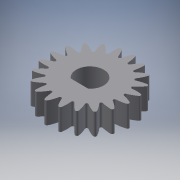
# Autodesk Inventor part: Kugg
Saved by Autodesk Inventor 2016 (Build 200138000, 138)
## iProperties
Created: 2018-03-02
Part Number: Kugg
Material: Generic
Document SubType Name: Modeling
Designer: Simon
Density: 1 g/cm^3
Appearance: Default
Author: Simon
Autodesk Inventor part; units mm, degrees
ref_plane "YZ Plane" through (0, 0, 0) normal (1, 0, 0) x (0, 1, 0)
ref_plane "XZ Plane" through (0, 0, 0) normal (0, 1, 0) x (-1, 0, 0)
ref_plane "XY Plane" through (0, 0, 0) normal (0, 0, 1) x (1, 0, 0)
sketch "Sketch1" plane through (0, 0, 0) normal (0, 0, 1) x (1, 0, 0)
  circle A0 centre (0, 0) radius 5.75
  arc A1 (0.266, 7.6325) -> (-0.3296, 5.7405) centre (6.5778, 4.6059) ccw
  arc A2 (1.143, 5.6352) -> (0.8227, 7.5927) centre (-5.8555, 5.495) ccw
  arc A3 (0.8227, 7.5927) -> (0.266, 7.6325) centre (0.5365, 7.5028) ccw
  arc A4 (-2.1056, 7.3412) -> (-2.0874, 5.3577) centre (4.8326, 6.4131) ccw
  arc A5 (-1.5638, 7.4753) -> (-2.1056, 7.3412) centre (-1.8082, 7.3014) ccw
  arc A6 (-0.6543, 5.7127) -> (-1.5638, 7.4753) centre (-7.267, 3.4166) ccw
  arc A7 (-4.2711, 6.3312) -> (-3.6408, 4.4505) centre (2.6143, 7.5926) ccw
  arc A8 (-3.7973, 6.6262) -> (-4.2711, 6.3312) centre (-3.976, 6.3853) ccw
  arc A9 (-2.3876, 5.2309) -> (-3.7973, 6.6262) centre (-7.9671, 1.0037) ccw
  arc A10 (-6.0185, 4.7015) -> (-4.8379, 3.1076) centre (0.1401, 8.0288) ccw
  arc A11 (-5.659, 5.1285) -> (-6.0185, 4.7015) centre (-5.7545, 4.8441) ccw
  arc A12 (-3.8871, 4.2371) -> (-5.659, 5.1285) centre (-7.8873, -1.5074) ccw
  arc A13 (-7.1768, 2.6116) -> (-5.5614, 1.4605) centre (-2.3478, 7.6792) ccw
  arc A14 (-6.9669, 3.1287) -> (-7.1768, 2.6116) centre (-6.9698, 2.8288) ccw
  arc A15 (-5.0062, 2.8285) -> (-6.9669, 3.1287) centre (-7.0355, -3.8709) ccw
  arc A16 (-7.6325, 0.266) -> (-5.7405, -0.3296) centre (-4.6059, 6.5778) ccw
  arc A17 (-7.5927, 0.8227) -> (-7.6325, 0.266) centre (-7.5028, 0.5365) ccw
  arc A18 (-5.6352, 1.143) -> (-7.5927, 0.8227) centre (-5.495, -5.8555) ccw
  arc A19 (-7.3412, -2.1056) -> (-5.3577, -2.0874) centre (-6.4131, 4.8326) ccw
  arc A20 (-7.4753, -1.5638) -> (-7.3412, -2.1056) centre (-7.3014, -1.8082) ccw
  arc A21 (-5.7127, -0.6543) -> (-7.4753, -1.5638) centre (-3.4166, -7.267) ccw
  arc A22 (-6.3312, -4.2711) -> (-4.4505, -3.6408) centre (-7.5926, 2.6143) ccw
  arc A23 (-6.6262, -3.7973) -> (-6.3312, -4.2711) centre (-6.3853, -3.976) ccw
  arc A24 (-5.2309, -2.3876) -> (-6.6262, -3.7973) centre (-1.0037, -7.9671) ccw
  arc A25 (-4.7015, -6.0185) -> (-3.1076, -4.8379) centre (-8.0288, 0.1401) ccw
  arc A26 (-5.1285, -5.659) -> (-4.7015, -6.0185) centre (-4.8441, -5.7545) ccw
  arc A27 (-4.2371, -3.8871) -> (-5.1285, -5.659) centre (1.5074, -7.8873) ccw
  arc A28 (-2.6116, -7.1768) -> (-1.4605, -5.5614) centre (-7.6792, -2.3478) ccw
  arc A29 (-3.1287, -6.9669) -> (-2.6116, -7.1768) centre (-2.8288, -6.9698) ccw
  arc A30 (-2.8285, -5.0062) -> (-3.1287, -6.9669) centre (3.8709, -7.0355) ccw
  arc A31 (-0.266, -7.6325) -> (0.3296, -5.7405) centre (-6.5778, -4.6059) ccw
  arc A32 (-0.8227, -7.5927) -> (-0.266, -7.6325) centre (-0.5365, -7.5028) ccw
  arc A33 (-1.143, -5.6352) -> (-0.8227, -7.5927) centre (5.8555, -5.495) ccw
  arc A34 (2.1056, -7.3412) -> (2.0874, -5.3577) centre (-4.8326, -6.4131) ccw
  arc A35 (1.5638, -7.4753) -> (2.1056, -7.3412) centre (1.8082, -7.3014) ccw
  arc A36 (0.6543, -5.7127) -> (1.5638, -7.4753) centre (7.267, -3.4166) ccw
  arc A37 (4.2711, -6.3312) -> (3.6408, -4.4505) centre (-2.6143, -7.5926) ccw
  arc A38 (3.7973, -6.6262) -> (4.2711, -6.3312) centre (3.976, -6.3853) ccw
  arc A39 (2.3876, -5.2309) -> (3.7973, -6.6262) centre (7.9671, -1.0037) ccw
  arc A40 (6.0185, -4.7015) -> (4.8379, -3.1076) centre (-0.1401, -8.0288) ccw
  arc A41 (5.659, -5.1285) -> (6.0185, -4.7015) centre (5.7545, -4.8441) ccw
  arc A42 (3.8871, -4.2371) -> (5.659, -5.1285) centre (7.8873, 1.5074) ccw
  arc A43 (7.1768, -2.6116) -> (5.5614, -1.4605) centre (2.3478, -7.6792) ccw
  arc A44 (6.9669, -3.1287) -> (7.1768, -2.6116) centre (6.9698, -2.8288) ccw
  arc A45 (5.0062, -2.8285) -> (6.9669, -3.1287) centre (7.0355, 3.8709) ccw
  arc A46 (7.6325, -0.266) -> (5.7405, 0.3296) centre (4.6059, -6.5778) ccw
  arc A47 (7.5927, -0.8227) -> (7.6325, -0.266) centre (7.5028, -0.5365) ccw
  arc A48 (5.6352, -1.143) -> (7.5927, -0.8227) centre (5.495, 5.8555) ccw
  arc A49 (7.3412, 2.1056) -> (5.3577, 2.0874) centre (6.4131, -4.8326) ccw
  arc A50 (7.4753, 1.5638) -> (7.3412, 2.1056) centre (7.3014, 1.8082) ccw
  arc A51 (5.7127, 0.6543) -> (7.4753, 1.5638) centre (3.4166, 7.267) ccw
  arc A52 (6.3312, 4.2711) -> (4.4505, 3.6408) centre (7.5926, -2.6143) ccw
  arc A53 (6.6262, 3.7973) -> (6.3312, 4.2711) centre (6.3853, 3.976) ccw
  arc A54 (5.2309, 2.3876) -> (6.6262, 3.7973) centre (1.0037, 7.9671) ccw
  arc A55 (4.7015, 6.0185) -> (3.1076, 4.8379) centre (8.0288, -0.1401) ccw
  arc A56 (5.1285, 5.659) -> (4.7015, 6.0185) centre (4.8441, 5.7545) ccw
  arc A57 (4.2371, 3.8871) -> (5.1285, 5.659) centre (-1.5074, 7.8873) ccw
  arc A58 (2.6116, 7.1768) -> (1.4605, 5.5614) centre (7.6792, 2.3478) ccw
  arc A59 (3.1287, 6.9669) -> (2.6116, 7.1768) centre (2.8288, 6.9698) ccw
  arc A60 (2.8285, 5.0062) -> (3.1287, 6.9669) centre (-3.8709, 7.0355) ccw
  arc A61 (0.6543, -5.7127) -> (2.0874, -5.3577) centre (0, 0) ccw
  arc A62 (2.3876, -5.2309) -> (3.6408, -4.4505) centre (0, 0) ccw
  arc A63 (3.8871, -4.2371) -> (4.8379, -3.1076) centre (0, 0) ccw
  arc A64 (5.0062, -2.8285) -> (5.5614, -1.4605) centre (0, 0) ccw
  arc A65 (5.6352, -1.143) -> (5.7405, 0.3296) centre (0, 0) ccw
  arc A66 (5.7127, 0.6543) -> (5.3577, 2.0874) centre (0, 0) ccw
  arc A67 (5.2309, 2.3876) -> (4.4505, 3.6408) centre (0, 0) ccw
  arc A68 (4.2371, 3.8871) -> (3.1076, 4.8379) centre (0, 0) ccw
  arc A69 (2.8285, 5.0062) -> (1.4605, 5.5614) centre (0, 0) ccw
  arc A70 (1.143, 5.6352) -> (-0.3296, 5.7405) centre (0, 0) ccw
  arc A71 (-0.6543, 5.7127) -> (-2.0874, 5.3577) centre (0, 0) ccw
  arc A72 (-2.3876, 5.2309) -> (-3.6408, 4.4505) centre (0, 0) ccw
  arc A73 (-3.8871, 4.2371) -> (-4.8379, 3.1076) centre (0, 0) ccw
  arc A74 (-5.0062, 2.8285) -> (-5.5614, 1.4605) centre (0, 0) ccw
  arc A75 (-5.6352, 1.143) -> (-5.7405, -0.3296) centre (0, 0) ccw
  arc A76 (-5.7127, -0.6543) -> (-5.3577, -2.0874) centre (0, 0) ccw
  arc A77 (-5.2309, -2.3876) -> (-4.4505, -3.6408) centre (0, 0) ccw
  arc A78 (-4.2371, -3.8871) -> (-3.1076, -4.8379) centre (0, 0) ccw
  arc A79 (-2.8285, -5.0062) -> (-1.4605, -5.5614) centre (0, 0) ccw
  arc A80 (-1.143, -5.6352) -> (0.3296, -5.7405) centre (0, 0) ccw
  point P0 (0, 7)
  point P1 (-2.1631, 6.6574)
  point P2 (-4.1145, 5.6631)
  point P3 (-5.6631, 4.1145)
  point P4 (-6.6574, 2.1631)
  point P5 (-7, 0)
  point P6 (-6.6574, -2.1631)
  point P7 (-5.6631, -4.1145)
  point P8 (-4.1145, -5.6631)
  point P9 (-2.1631, -6.6574)
  point P10 (0, -7)
  point P11 (2.1631, -6.6574)
  point P12 (4.1145, -5.6631)
  point P13 (5.6631, -4.1145)
  point P14 (6.6574, -2.1631)
  point P15 (7, 0)
  point P16 (6.6574, 2.1631)
  point P17 (5.6631, 4.1145)
  point P18 (4.1145, 5.6631)
  point P19 (2.1631, 6.6574)
  dimension "d12" = 0.3
  dimension "d17" = 360
  dimension "d21" = 360
  constraints: 180 point on circle, 80 centre point, 2 tangent, 306 other
  measures "d12" radius of A3
sketch "Sketch4" plane through (0, 0, 0) normal (0, 0, 1) x (1, 0, 0)
  circle A0 centre (0, 0) radius 5.75
  arc A1 (0.266, 7.6325) -> (-0.3296, 5.7405) centre (6.5778, 4.6059) ccw projected
  arc A2 (0.8227, 7.5927) -> (0.266, 7.6325) centre (0.5365, 7.5028) ccw projected
  arc A3 (1.143, 5.6352) -> (0.8227, 7.5927) centre (-5.8555, 5.495) ccw projected
  arc A4 (0, 7) -> (-0.3296, 5.7405) centre (6.5778, 4.6059) ccw
  arc A5 (1.143, 5.6352) -> (0.9807, 7) centre (-5.8555, 5.495) ccw
  arc A6 (0.266, 7.6325) -> (0, 7) centre (6.5778, 4.6059) ccw
  arc A7 (0.9807, 7) -> (0.8227, 7.5927) centre (-5.8555, 5.495) ccw
  arc A8 (0.8227, 7.5927) -> (0.266, 7.6325) centre (0.5365, 7.5028) ccw
  dimension "d23" = 11.5
  constraints: 12 point on circle, 5 centre point, 2 concentric, 1 coincident, 3 other
extrude "Extrusion2" add sketch "Sketch4" along normal blind 4 contours A0
sketch "Sketch5" plane through (0, 0, 0) normal (0, 0, -1) x (-1, 0, 0)
  arc A0 (-0.9807, 7) -> (-1.143, 5.6352) centre (5.8555, 5.495) ccw projected
  arc A1 (-0.8227, 7.5927) -> (-1.143, 5.6352) centre (5.8555, 5.495) ccw projected
  arc A2 (-0.266, 7.6325) -> (-0.8227, 7.5927) centre (-0.5365, 7.5028) ccw projected
  arc A3 (0, 7) -> (-0.266, 7.6325) centre (-6.5778, 4.6059) ccw projected
  arc A4 (0.3296, 5.7405) -> (-0.266, 7.6325) centre (-6.5778, 4.6059) ccw projected
  arc A5 (0.3296, 5.7405) -> (-1.143, 5.6352) centre (0, 0) ccw
  point P0 (0, 0)
  constraints: 2 point on circle, 1 centre point
extrude "Extrusion3" add sketch "Sketch5" against normal blind 4
pattern_circular "Circular Pattern1" count 20 over 360 about axis through (0, 0, -10) along (0, 0, 1) of "Extrusion3"
fillet "Fillet2" radius 0.25 40 edges at (1.143, 5.6352, 2) (1.4605, 5.5614, 2) (2.8285, 5.0062, 2) (3.1076, 4.8379, 2) (4.2371, 3.8871, 2) (4.4505, 3.6408, 2) (5.2309, 2.3876, 2) (5.3577, 2.0874, 2) (5.7127, 0.6543, 2) (5.7405, 0.3296, 2) (5.6352, -1.143, 2) (5.5614, -1.4605, 2) (5.0062, -2.8285, 2) (4.8379, -3.1076, 2) (3.8871, -4.2371, 2) (3.6408, -4.4505, 2) (2.3876, -5.2309, 2) (2.0874, -5.3577, 2) (0.6543, -5.7127, 2) (0.3296, -5.7405, 2) (-1.143, -5.6352, 2) (-1.4605, -5.5614, 2) (-2.8285, -5.0062, 2) (-3.1076, -4.8379, 2) (-4.2371, -3.8871, 2) (-4.4505, -3.6408, 2) (-5.2309, -2.3876, 2) (-5.3577, -2.0874, 2) (-5.7127, -0.6543, 2) (-5.7405, -0.3296, 2) (-5.6352, 1.143, 2) (-5.5614, 1.4605, 2) (-5.0062, 2.8285, 2) (-4.8379, 3.1076, 2) (-3.8871, 4.2371, 2) (-3.6408, 4.4505, 2) (-2.3876, 5.2309, 2) (-2.0874, 5.3577, 2) (-0.6543, 5.7127, 2) (-0.3296, 5.7405, 2)
sketch "Sketch6" plane through (0, 0, 0) normal (0, 0, -1) x (-1, 0, 0)
  line L0 (-1.6432, -1.95) -> (1.6667, -1.9299)
  arc A0 (1.6667, -1.9299) -> (-1.6432, -1.95) centre (0, 0) ccw
  dimension "d38" = 2.55
  dimension "d39" = 1.94
  constraints: 2 end point, 2 point on circle, 1 centre point, 1 coincident
  measures "d38" radius of A0
  measures "d39" distance from line of point (0, 0) L0
extrude "Extrusion4" cut sketch "Sketch6" against normal through all
body "Solid2"
